Autodesk Fusion 360 part; units mm, degrees
(part 2 of 2)
sketch "Sketch37" plane through (0, 0, 85) normal (0, 0, 1) x (-1, 0, 0) in component "Boden"
  line L0 (-120.5, -36) -> (-120.5, -2.5)
  line L1 (-120.5, -2.5) -> (-127.5, -2.5)
  line L2 (-127.5, -2.5) -> (-127.5, -36)
  line L3 (-127.5, -36) -> (-120.5, -36)
  circle A0 centre (-124, -29.5) radius 1.75
  circle A1 centre (-124, -9) radius 1.75
  circle A2 centre (-169, -29.5) radius 1.75
  circle A3 centre (-169, -9) radius 1.75
  line L4 (-120.5, -33) -> (-127.5, -33)
  line L5 (-172.5, -2.5) -> (-172.5, -36)
  line L6 (-127.5, -5.5) -> (-120.5, -5.5)
  dimension "d285" = 3.5
  dimension "d286" = 7
  dimension "d287" = 3.5
  dimension "d288" = 3.5
  dimension "d289" = 3.5
  dimension "d290" = 3.5
  constraint vertical A0.centre A1.centre
  constraint horizontal A1.centre A3.centre
  constraint vertical A2.centre A3.centre
  constraint horizontal A0.centre A2.centre
  constraint equal A0 A1
  constraint equal A1 A3
  constraint equal A2 A3
  measures "d285" distance of L0 A0.centre
  measures "d286" distance of L0.start L2.end
  measures "d287" distance of A0.centre L4
  measures "d288" distance of A2.centre L5
  measures "d289" distance of A1.centre L6
  measures "d290" diameter of A0
extrude "Extrude43" cut sketch "Sketch37" against normal up to surface (3 mm away) contours A0 | A1 | A2 | A3 bodies 1 in component "Boden"
sketch "Sketch1 (2)" plane through (0, 0, 85) normal (0, 0, 1) x (-1, 0, 0) in component "Pins"
  circle A0 centre (-124, -29.5) radius 1.75
  circle A1 centre (-124, -9) radius 1.75
  line L0 (-120.5, -36) -> (-120.5, -2.5)
  line L1 (-120.5, -2.5) -> (-127.5, -2.5)
  line L2 (-127.5, -2.5) -> (-127.5, -36) construction
  line L3 (-127.5, -36) -> (-120.5, -36)
  line L4 (-172.5, -36) -> (-172.5, -2.5)
  line L5 (-172.5, -2.5) -> (-120.5, -2.5)
  line L6 (-120.5, -2.5) -> (-120.5, -36)
  line L7 (-172.5, -2.5) -> (-172.5, -36)
  circle A2 centre (-169, -29.5) radius 1.75
  circle A3 centre (-169, -9) radius 1.75
  line L8 (-150.5, -36) -> (-150.5, -50)
  line L9 (-150.5, -50) -> (-132.5, -50)
  line L10 (-132.5, -50) -> (-132.5, -36)
  line L11 (-120.5, -36) -> (-132.5, -36)
  line L12 (-150.5, -36) -> (-172.5, -36)
  dimension "d332" = 14
  dimension "d333" = 18
  dimension "d334" = 22
  constraint horizontal L11
  constraint vertical L4
  constraint horizontal L5
  constraint vertical L6
  constraint collinear L0 L6
  constraint collinear L4 L7
  constraint collinear L1 L5
  constraint collinear L3 L11
  constraint vertical L8
  constraint horizontal L9
  constraint vertical L10
  constraint collinear L11 L12
  measures "d332" distance of L10.end L9.end
  measures "d333" distance of L8.end L9.end
  measures "d334" distance of L4 L8
extrude "Extrude1''" add sketch "Sketch1 (2)" along normal blind 3 separate body makes body 3 in component "Pins"
sketch "Sketch2" plane through (0, 0, 85) normal (0, 0, -1) x (1, 0, 0) in component "Pins"
  circle A0 centre (169, -9) radius 1.75
  circle A1 centre (124, -29.5) radius 1.75
  circle A2 centre (124, -9) radius 1.75
  circle A3 centre (169, -29.5) radius 1.75
  line L0 (172.5, -2.5) -> (120.5, -2.5)
  line L1 (120.5, -2.5) -> (120.5, -36)
  line L2 (150.5, -36) -> (172.5, -36)
  line L3 (172.5, -36) -> (172.5, -2.5)
  line L4 (161.1, -8.85) -> (155.6, -8.85)
  line L5 (155.6, -8.85) -> (155.6, -6.15)
  line L6 (155.6, -6.15) -> (161.1, -6.15)
  line L7 (161.1, -6.15) -> (161.1, -8.85)
  line L8 (161.1, -10.85) -> (161.1, -13.55)
  line L9 (155.6, -13.55) -> (155.6, -10.85)
  line L10 (155.6, -10.85) -> (161.1, -10.85)
  line L11 (161.1, -13.55) -> (155.6, -13.55)
  line L12 (161.1, -15.55) -> (161.1, -18.25)
  line L13 (155.6, -18.25) -> (155.6, -15.55)
  line L14 (155.6, -15.55) -> (161.1, -15.55)
  line L15 (161.1, -18.25) -> (155.6, -18.25)
  line L16 (161.1, -20.25) -> (161.1, -22.95)
  line L17 (155.6, -22.95) -> (155.6, -20.25)
  line L18 (155.6, -20.25) -> (161.1, -20.25)
  line L19 (161.1, -22.95) -> (155.6, -22.95)
  line L20 (161.1, -24.95) -> (161.1, -27.65)
  line L21 (155.6, -27.65) -> (155.6, -24.95)
  line L22 (155.6, -24.95) -> (161.1, -24.95)
  line L23 (161.1, -27.65) -> (155.6, -27.65)
  line L24 (155.6, -29.65) -> (161.1, -29.65)
  line L25 (155.6, -32.35) -> (155.6, -29.65)
  line L26 (161.1, -32.35) -> (155.6, -32.35)
  line L27 (161.1, -29.65) -> (161.1, -32.35)
  line L28 (150.6, -8.85) -> (142.4, -8.85)
  line L29 (142.4, -8.85) -> (142.4, -6.15)
  line L30 (142.4, -6.15) -> (150.6, -6.15)
  line L31 (150.6, -6.15) -> (150.6, -8.85)
  line L32 (165.5, -33) -> (165.5, -5.5)
  line L33 (142.4, -10.85) -> (150.6, -10.85)
  line L34 (150.6, -10.85) -> (150.6, -13.55)
  line L35 (150.6, -13.55) -> (142.4, -13.55)
  line L36 (142.4, -13.55) -> (142.4, -10.85)
  line L37 (142.4, -15.55) -> (150.6, -15.55)
  line L38 (150.6, -15.55) -> (150.6, -18.25)
  line L39 (150.6, -18.25) -> (142.4, -18.25)
  line L40 (142.4, -18.25) -> (142.4, -15.55)
  line L41 (142.4, -20.25) -> (150.6, -20.25)
  line L42 (150.6, -20.25) -> (150.6, -22.95)
  line L43 (150.6, -22.95) -> (142.4, -22.95)
  line L44 (142.4, -22.95) -> (142.4, -20.25)
  line L45 (137.4, -8.85) -> (131.9, -8.85)
  line L46 (131.9, -8.85) -> (131.9, -6.15)
  line L47 (131.9, -6.15) -> (137.4, -6.15)
  line L48 (137.4, -6.15) -> (137.4, -8.85)
  line L49 (137.4, -10.85) -> (137.4, -13.55)
  line L50 (131.9, -10.85) -> (137.4, -10.85)
  line L51 (131.9, -13.55) -> (131.9, -10.85)
  line L52 (137.4, -13.55) -> (131.9, -13.55)
  line L53 (137.4, -15.55) -> (137.4, -18.25)
  line L54 (131.9, -15.55) -> (137.4, -15.55)
  line L55 (131.9, -18.25) -> (131.9, -15.55)
  line L56 (137.4, -18.25) -> (131.9, -18.25)
  line L57 (137.4, -20.25) -> (137.4, -22.95)
  line L58 (131.9, -20.25) -> (137.4, -20.25)
  line L59 (131.9, -22.95) -> (131.9, -20.25)
  line L60 (137.4, -22.95) -> (131.9, -22.95)
  line L61 (142.5, -31) -> (137, -31)
  line L62 (137, -31) -> (137, -28.3)
  line L63 (137, -28.3) -> (142.5, -28.3)
  line L64 (142.5, -28.3) -> (142.5, -31)
  line L65 (132.5, -50) -> (150.5, -50)
  line L66 (150.5, -50) -> (150.5, -36)
  line L67 (120.5, -36) -> (132.5, -36)
  line L68 (132.5, -36) -> (132.5, -50)
  line L69 (139.35, -47) -> (143.65, -47)
  line L70 (146.65, -44) -> (146.65, -40)
  line L71 (143.65, -37) -> (139.35, -37)
  line L72 (136.35, -40) -> (136.35, -44)
  line L73 (130.9, -23.95) -> (138.4, -23.95)
  line L74 (138.4, -23.95) -> (138.4, -5.15)
  line L75 (138.4, -5.15) -> (130.9, -5.15)
  line L76 (130.9, -5.15) -> (130.9, -23.95)
  line L77 (141.4, -23.95) -> (151.6, -23.95)
  line L78 (151.6, -23.95) -> (151.6, -5.15)
  line L79 (151.6, -5.15) -> (141.4, -5.15)
  line L80 (141.4, -5.15) -> (141.4, -23.95)
  line L81 (154.6, -5.15) -> (162.1, -5.15)
  line L82 (162.1, -5.15) -> (162.1, -33.35)
  line L83 (162.1, -33.35) -> (154.6, -33.35)
  line L84 (154.6, -33.35) -> (154.6, -5.15)
  line L85 (136, -32) -> (143.5, -32)
  line L86 (143.5, -32) -> (143.5, -27.3)
  line L87 (143.5, -27.3) -> (136, -27.3)
  line L88 (136, -27.3) -> (136, -32)
  arc A4 (136.35, -44) -> (139.35, -47) centre (139.35, -44) ccw
  arc A5 (143.65, -47) -> (146.65, -44) centre (143.65, -44) ccw
  arc A6 (146.65, -40) -> (143.65, -37) centre (143.65, -40) ccw
  arc A7 (139.35, -37) -> (136.35, -40) centre (139.35, -40) ccw
  point P0 (136.35, -47)
  point P1 (146.65, -47)
  point P2 (136.35, -37)
  dimension "d295" = 5.5
  dimension "d296" = 2.7
  dimension "d297" = 3.65
  dimension "d298" = 7.9
  dimension "d300" = 2.7
  dimension "d302" = 2.7
  dimension "d304" = 2.7
  dimension "d306" = 2.7
  dimension "d307" = 2
  dimension "d308" = 2
  dimension "d309" = 2
  dimension "d310" = 2
  dimension "d311" = 2.7
  dimension "d312" = 2
  dimension "d313" = 3
  dimension "d314" = 8.2
  dimension "d316" = 5
  dimension "d317" = 1.5
  dimension "d324" = 5.5
  dimension "d326" = 5
  dimension "d330" = 5.5
  dimension "d331" = 2.7
  dimension "d335" = 4.5
  dimension "d336" = 4.3288
  dimension "d337" = 5
  dimension "d338" = 10.3
  dimension "d339" = 10
  dimension "d340" = 3.85
  dimension "d341" = 1.8
  dimension "d342" = 3
  dimension "d343" = 1
  dimension "d344" = 1
  dimension "d345" = 1
  dimension "d346" = 1
  dimension "d347" = 1
  dimension "d348" = 1
  dimension "d349" = 1
  dimension "d350" = 1
  dimension "d351" = 1
  dimension "d352" = 1
  dimension "d353" = 1
  dimension "d354" = 1
  dimension "d355" = 1
  dimension "d356" = 1
  dimension "d357" = 1
  dimension "d358" = 1
  dimension "d359" = 3
  dimension "d360" = 3
  dimension "d361" = 3
  dimension "d366" = 8.8
  constraint horizontal L4
  constraint vertical L5
  constraint horizontal L6
  constraint vertical L7
  constraint horizontal L11
  constraint vertical L9
  constraint horizontal L10
  constraint vertical L8
  constraint horizontal L15
  constraint vertical L13
  constraint horizontal L14
  constraint vertical L12
  constraint horizontal L19
  constraint vertical L17
  constraint horizontal L18
  constraint vertical L16
  constraint horizontal L23
  constraint vertical L21
  constraint horizontal L22
  constraint vertical L20
  constraint collinear L7 L8
  constraint collinear L8 L12
  constraint collinear L12 L16
  constraint collinear L16 L20
  constraint collinear L5 L9
  constraint collinear L9 L13
  constraint collinear L13 L17
  constraint collinear L17 L21
  constraint horizontal L26
  constraint vertical L25
  constraint horizontal L24
  constraint vertical L27
  constraint collinear L20 L27
  constraint collinear L21 L25
  constraint horizontal L28
  constraint vertical L29
  constraint horizontal L30
  constraint vertical L31
  constraint collinear L4 L28
  constraint horizontal L35
  constraint vertical L36
  constraint horizontal L33
  constraint vertical L34
  constraint horizontal L39
  constraint vertical L40
  constraint horizontal L37
  constraint vertical L38
  constraint horizontal L43
  constraint vertical L44
  constraint horizontal L41
  constraint vertical L42
  constraint collinear L29 L36
  constraint collinear L36 L40
  constraint collinear L40 L44
  constraint collinear L38 L42
  constraint collinear L34 L38
  constraint collinear L31 L34
  constraint collinear L6 L30
  constraint collinear L10 L33
  constraint collinear L11 L35
  constraint collinear L14 L37
  constraint collinear L15 L39
  constraint collinear L18 L41
  constraint collinear L19 L43
  constraint horizontal L45
  constraint vertical L46
  constraint horizontal L47
  constraint vertical L48
  constraint collinear L30 L47
  constraint collinear L28 L45
  constraint horizontal L52
  constraint vertical L51
  constraint horizontal L50
  constraint vertical L49
  constraint horizontal L56
  constraint vertical L55
  constraint horizontal L54
  constraint vertical L53
  constraint horizontal L60
  constraint vertical L59
  constraint horizontal L58
  constraint vertical L57
  constraint collinear L46 L51
  constraint collinear L51 L55
  constraint collinear L55 L59
  constraint collinear L53 L57
  constraint collinear L49 L53
  constraint collinear L48 L49
  constraint collinear L33 L50
  constraint collinear L35 L52
  constraint collinear L37 L54
  constraint collinear L39 L56
  constraint collinear L41 L58
  constraint collinear L43 L60
  constraint horizontal L61
  constraint vertical L62
  constraint horizontal L63
  constraint vertical L64
  constraint horizontal L69
  constraint vertical L70
  constraint horizontal L71
  constraint vertical L72
  constraint horizontal L73
  constraint vertical L74
  constraint horizontal L75
  constraint vertical L76
  constraint horizontal L77
  constraint vertical L78
  constraint horizontal L79
  constraint vertical L80
  constraint horizontal L81
  constraint vertical L82
  constraint horizontal L83
  constraint vertical L84
  constraint horizontal L85
  constraint vertical L86
  constraint horizontal L87
  constraint vertical L88
  constraint coincident P0 L69
  constraint coincident P0 L72
  constraint tangent L69 A4
  constraint tangent L72 A4
  constraint coincident P1 L69
  constraint coincident P1 L70
  constraint tangent L69 A5
  constraint tangent L70 A5
  constraint tangent L70 A6
  constraint tangent L71 A6
  constraint coincident P2 L71
  constraint coincident P2 L72
  constraint tangent L71 A7
  constraint tangent L72 A7
  constraint equal A6 A7
  measures "d295" distance of L4.start L4.end
  measures "d296" distance of L4.start L6.end
  measures "d297" distance of L0 L6
  measures "d298" distance of A0.centre L7
  measures "d300" distance of L8.end L8.start
  measures "d302" distance of L12.end L12.start
  measures "d304" distance of L16.end L16.start
  measures "d306" distance of L20.end L20.start
  measures "d307" distance of L4 L10
  measures "d308" distance of L11 L14
  measures "d309" distance of L15 L18
  measures "d310" distance of L19 L22
  measures "d311" distance of L26.start L24.end
  measures "d312" distance of L23 L24
  measures "d314" distance of L28.start L28.end
  measures "d316" distance of L5 L31
  measures "d324" distance of L45.start L45.end
  measures "d326" distance of L29 L48
  measures "d330" distance of L61.start L61.end
  measures "d331" distance of L61.start L63.end
  measures "d335" distance of L62 L68
  measures "d337" distance of L2 L61
  measures "d338" distance of P0 P1
  measures "d339" distance of P0 P2
  measures "d340" distance of L68 L72
  measures "d342" distance of L65 L69
  measures "d343" distance of L60 L73
  measures "d344" distance of L59 L76
  measures "d345" distance of L57 L74
  measures "d346" distance of L62 L88
  measures "d347" distance of L63 L87
  measures "d348" distance of L64 L86
  measures "d349" distance of L61 L85
  measures "d350" distance of L44 L80
  measures "d351" distance of L42 L78
  measures "d352" distance of L43 L77
  measures "d353" distance of L47 L75
  measures "d354" distance of L30 L79
  measures "d355" distance of L6 L81
  measures "d356" distance of L25 L84
  measures "d357" distance of L26 L83
  measures "d358" distance of L27 L82
  measures "d359" radius of A4
  measures "d360" radius of A5
  measures "d361" radius of A6
extrude "Extrude2'" add sketch "Sketch2" along normal blind 1.5 contours L73 L74 L75 L76 | L77 L78 L79 L80 | L81 L82 L83 L84 | L85 L86 L87 L88 bodies 3 in component "Pins"
extrude "Extrude3" cut sketch "Sketch2" against normal up to surface (3 mm away) contours L4 L5 L6 L7 | L8 L9 L10 L11 | L12 L13 L14 L15 | L16 L17 L18 L19 | L20 L21 L22 L23 | L24 L25 L26 L27 | L28 L29 L30 L31 | L33 L34 L35 L36 | L37 L38 L39 L40 | L41 L42 L43 L44 | L45 L46 L47 L48 | L49 L50 L51 L52 | L53 L54 L55 L56 | L57 L58 L59 L60 | L61 L62 L63 L64 | L69 L70 L71 L72 A4 A5 A6 A7 bodies 3 in component "Pins"
component "Boden" placed x (1, 0, 0) y (0, 1, 0) z (0, 0, 1) at (0, 0, 0)
component "Stromanschluss" placed x (1, 0, 0) y (0, 1, 0) z (0, 0, 1) at (0, 0, 0)
component "Pins" placed x (1, 0, 0) y (0, 1, 0) z (0, 0, 1) at (0, 0, 0)
equation "shell_thickness = 2.5 mm"
equation "d10 = 53 mm - d8"
equation "d14 = shell_thickness"
equation "d15 = shell_thickness"
equation "d20 = shell_thickness"
equation "d21 = shell_thickness"
equation "d22 = shell_thickness"
equation "d48 = shell_thickness"
equation "d50 = shell_thickness"
equation "d56 = shell_thickness"
equation "d57 = shell_thickness"
equation "d58 = shell_thickness"
equation "d70 = shell_thickness"
equation "d71 = shell_thickness"
equation "d74 = -shell_thickness"
equation "d78 = shell_thickness"
equation "d81 = -shell_thickness"
equation "d84 = shell_thickness"
equation "d85 = shell_thickness"
equation "d97 = d96"
equation "d99 = d98"
equation "d103 = -shell_thickness"
equation "d109 = shell_thickness"
equation "d115 = d114"
equation "d116 = d114"
equation "d117 = d114"
equation "d118 = shell_thickness"
equation "d123 = d122"
equation "d126 = shell_thickness"
equation "d127 = shell_thickness"
equation "d128 = shell_thickness"
equation "d136 = shell_thickness"
equation "d137 = shell_thickness"
equation "d140 = d135"
equation "d141 = d138"
equation "d142 = shell_thickness"
equation "d143 = shell_thickness"
equation "d148 = shell_thickness"
equation "d150 = shell_thickness"
equation "d159 = d158"
equation "d160 = d158"
equation "d161 = d158"
equation "d192 = d190"
equation "d193 = d191"
equation "d194 = d190"
equation "d196 = d191"
equation "d265 = shell_thickness"
equation "d284 = -shell_thickness / 2"
equation "d287 = d285"
equation "d288 = d285"
equation "d289 = d285"
equation "d295 = d324"
equation "d300 = d296"
equation "d302 = d296"
equation "d304 = d296"
equation "d306 = d296"
equation "d308 = d307"
equation "d309 = d307"
equation "d310 = d307"
equation "d311 = d296"
equation "d312 = d307"
equation "d326 = d316"
equation "d330 = d324"
equation "d331 = d296"
equation "d344 = d343"
equation "d345 = d343"
equation "d346 = d343"
equation "d347 = d343"
equation "d348 = d343"
equation "d349 = d343"
equation "d350 = d343"
equation "d351 = d343"
equation "d352 = d343"
equation "d353 = d343"
equation "d354 = d343"
equation "d355 = d343"
equation "d356 = d343"
equation "d357 = d343"
equation "d358 = d343"
equation "d360 = d359"
equation "d361 = d359"
